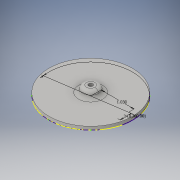
# Autodesk Inventor part: small encoder wheel noah 1
Saved by Autodesk Inventor 2016 (Build 200138000, 138)
## iProperties
Created: 2016-12-02
Part Number: small encoder wheel noah 1
Material: Generic
Document SubType Name: Modeling
Designer: Student
Density: 1 g/cm^3
Appearance: Default
Author: Student
Autodesk Inventor part; units mm, degrees
ref_plane "YZ Plane" through (0, 0, 0) normal (1, 0, 0) x (0, 1, 0)
ref_plane "XZ Plane" through (0, 0, 0) normal (0, 1, 0) x (-1, 0, 0)
ref_plane "XY Plane" through (0, 0, 0) normal (0, 0, 1) x (1, 0, 0)
sketch "Sketch1" plane through (0, 0, 0) normal (0, 1, 0) x (-1, 0, 0)
  circle A0 centre (0, 0) radius 33.02
  dimension "d0" = 66.04
  constraints: 1 centre point, 1 coincident
  measures "d0" diameter of A0
extrude "Extrusion1" add sketch "Sketch1" along normal blind 2.54
sketch "Sketch2" plane through (0, 2.54, 0) normal (0, 1, 0) x (1, 0, 0)
  circle A0 centre (0, 0) radius 6.35
  dimension "d4" = 12.7
  constraints: 1 centre point, 1 coincident
  measures "d4" diameter of A0
extrude "Extrusion2" add sketch "Sketch2" along normal blind 5.08
fillet "Fillet1" radius 3.175 1 edges at (-6.35, 2.54, 0)
sketch "Sketch3" plane through (0, 7.62, 0) normal (0, 1, 0) x (1, 0, 0)
  circle A0 centre (0, 0) radius 1.6637
  dimension "d8" = 3.3274
  constraints: 1 centre point, 1 coincident
  measures "d8" diameter of A0
extrude "Extrusion3" cut sketch "Sketch3" against normal blind 7.62
fillet "Fillet2" radius 3.175 1 edges at (-6.35, 7.62, 0)
sketch "Sketch4" plane through (0, 0, 0) normal (0, -1, 0) x (1, 0, 0)
  point P0 (0, 0)
sketch "Sketch7" plane through (0, 0, 0) normal (0, -1, 0) x (1, 0, 0)
  circle A0 centre (0, 0) radius 33.02 projected
  arc A1 (32.1408, -7.5691) -> (33.02, 0) centre (0, 0) ccw
  arc A2 (33.02, 0) -> (32.1572, 7.4991) centre (0, 0) ccw
  circle A3 centre (0, 0) radius 1.6637 projected
  line L0 (0, 0) -> (32.6627, -4.8446)
  line L1 (0, 0) -> (32.4709, 5.9969)
  arc A4 (32.6627, -4.8446) -> (32.4709, 5.9969) centre (0, 0) ccw
  line L2 (26.162, -3.8804) -> (26.162, 4.8318)
  arc A5 (32.6627, -4.8446) -> (32.4709, 5.9969) centre (0, 0) ccw
  arc A6 (26.5217, 19.6703) -> (18.7199, 27.2008) centre (0, 0) ccw
  line L3 (0, 0) -> (26.5217, 19.6703)
  line L4 (21.2432, 15.7555) -> (15.0827, 21.9159)
  line L5 (0, 0) -> (18.7199, 27.2008)
  arc A7 (4.8446, 32.6627) -> (-5.9969, 32.4709) centre (0, 0) ccw
  line L6 (0, 0) -> (4.8446, 32.6627)
  line L7 (3.8804, 26.162) -> (-4.8318, 26.162)
  line L8 (0, 0) -> (-5.9969, 32.4709)
  arc A8 (-19.6703, 26.5217) -> (-27.2008, 18.7199) centre (0, 0) ccw
  line L9 (0, 0) -> (-19.6703, 26.5217)
  line L10 (-15.7555, 21.2432) -> (-21.9159, 15.0827)
  line L11 (0, 0) -> (-27.2008, 18.7199)
  arc A9 (-32.6627, 4.8446) -> (-32.4709, -5.9969) centre (0, 0) ccw
  line L12 (0, 0) -> (-32.6627, 4.8446)
  line L13 (-26.162, 3.8804) -> (-26.162, -4.8318)
  line L14 (0, 0) -> (-32.4709, -5.9969)
  arc A10 (-26.5217, -19.6703) -> (-18.7199, -27.2008) centre (0, 0) ccw
  line L15 (0, 0) -> (-26.5217, -19.6703)
  line L16 (-21.2432, -15.7555) -> (-15.0827, -21.9159)
  line L17 (0, 0) -> (-18.7199, -27.2008)
  arc A11 (-4.8446, -32.6627) -> (5.9969, -32.4709) centre (0, 0) ccw
  line L18 (0, 0) -> (-4.8446, -32.6627)
  line L19 (-3.8804, -26.162) -> (4.8318, -26.162)
  line L20 (0, 0) -> (5.9969, -32.4709)
  arc A12 (19.6703, -26.5217) -> (27.2008, -18.7199) centre (0, 0) ccw
  line L21 (0, 0) -> (19.6703, -26.5217)
  line L22 (15.7555, -21.2432) -> (21.9159, -15.0827)
  line L23 (0, 0) -> (27.2008, -18.7199)
  point P0 (23.3487, 23.3487)
  point P1 (0, 33.02)
  point P2 (-23.3487, 23.3487)
  point P3 (-33.02, 0)
  point P4 (-23.3487, -23.3487)
  point P5 (0, -33.02)
  point P6 (23.3487, -23.3487)
  dimension "d25" = 26.162
  dimension "d26" = 8.7122
  dimension "d29" = 360
  constraints: 48 end point, 38 point on circle, 16 point on line, 11 centre point, 1 concentric, 1 vertical, 89 other
  measures "d25" distance from line of point (0, 0) L2
  measures "d26" distance of L2.start L2.end
body "Solid1"
